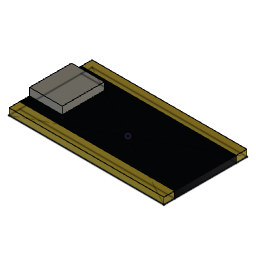
nice!nano v1.0 holder v25 (Autodesk Fusion 360 archive; units mm, degrees)
design "nice!nano v1.0"
Autodesk Fusion 360 part; units mm, degrees
sketch "pcb" plane through (0, 0, 0) normal (0, 0, 1) x (1, 0, 0)
  line L0 (16.6, -8.9) -> (-16.6, -8.9)
  line L1 (-16.6, -8.9) -> (-16.6, 8.9)
  line L2 (-16.6, 8.9) -> (16.6, 8.9)
  line L3 (16.6, 8.9) -> (16.6, -8.9)
  line L4 (16.6, -8.9) -> (-16.6, 8.9) construction
  line L5 (-16.6, -8.9) -> (16.6, 8.9) construction
  line L6 (-16.6, -6.6) -> (16.6, -6.6)
  line L7 (-16.6, 6.6) -> (16.6, 6.6)
  dimension "d7" = 33.2
  dimension "d8" = 17.8
  dimension "d18" = 2.3
  dimension "d20" = 2.3
  constraint horizontal L0
  constraint perpendicular L0 L1
  constraint parallel L0 L2
  constraint parallel L1 L3
  constraint coincident L4 origin
  constraint coincident L5 origin
  constraint coincident L1 L6.start
  constraint coincident L3 L6.end
  constraint perpendicular L3 L6
  constraint coincident L1 L7.start
  constraint coincident L3 L7.end
  constraint perpendicular L3 L7
  measures "d7" distance of L1.end L2.end
  measures "d8" distance of L0.end L1.end
  measures "d18" distance of L0 L6
  measures "d20" distance of L2.end L7.end
extrude "Extrude1" add sketch "pcb" along normal blind 1.4 makes body 1
sketch "usb" plane through (0, 0, 0) normal (0, 0, 1) x (1, 0, 0)
  line L0 (-16.6, -4.5) -> (-9.6, -4.5)
  line L1 (-9.6, -4.5) -> (-9.6, 4.5)
  line L2 (-9.6, 4.5) -> (-16.6, 4.5)
  line L3 (-16.6, 4.5) -> (-16.6, -4.5)
  line L4 (-16.6, 8.9) -> (-16.6, -8.9)
  dimension "d11" = 7
  dimension "d12" = 9
  dimension "d13" = 4.4
  constraint horizontal L0
  constraint vertical L1
  constraint horizontal L2
  constraint vertical L3
  constraint coincident L0.start L4
  measures "d11" distance of L0.start L0.end
  measures "d12" distance of L0.start L2.end
  measures "d13" distance of L0.start L4.end
extrude "Extrude2" cut sketch "usb" along normal blind 3 bodies 1
extrude "Extrude3" add sketch "usb" along normal blind 3 separate body makes body 2
extrude "Extrude4" add sketch "pcb" along normal blind 1.4 separate body contours L0 L1 L3 L6 makes body 3
extrude "Extrude5" cut sketch "pcb" along normal blind 1.4 contours L1 L2 L3 L7 bodies 1
extrude "Extrude6" add sketch "pcb" along normal blind 1.4 separate body contours L1 L2 L3 L7 makes body 4
extrude "Extrude7" cut sketch "pcb" along normal blind 1.4 contours L0 L1 L3 L6 bodies 1
copy_body "Body->Comp1" bodies 1 removing the originals makes body 5 in component "nice!nano v1.0"
copy_body "CutPasteBodies4" bodies 2 removing the originals makes body 6 in component "nice!nano v1.0"
copy_body "CutPasteBodies5" bodies 4 removing the originals makes body 7 in component "nice!nano v1.0"
copy_body "CutPasteBodies6" bodies 3 removing the originals makes body 8 in component "nice!nano v1.0"
component "nice!nano v1.0" placed x (1, 0, 0) y (0, 1, 0) z (0, 0, 1) at (0, 0, 0)
equation "length = 33.2 mm"
equation "width = 17.8 mm"
equation "height = 1.4 mm"
equation "usbWidth = 9 mm"
equation "usbHeight = 3 mm"
equation "usbDepth = 7 mm"
equation "d7 = length"
equation "d8 = width"
equation "d9 = height"
equation "d11 = usbDepth"
equation "d12 = usbWidth"
equation "d13 = ( width - usbWidth ) / 2"
equation "d14 = usbHeight"
equation "d16 = usbHeight"
equation "d18 = headerWidth"
equation "headerWidth = 2.3 mm"
equation "d20 = headerWidth"
equation "d21 = height"
equation "d23 = height"
equation "d25 = height"
equation "d27 = height"
named bodies: "pcb", "usb", "gpio1", "gpio2", "usb (1)", "gpio2 (1)", "gpio1 (1)"
